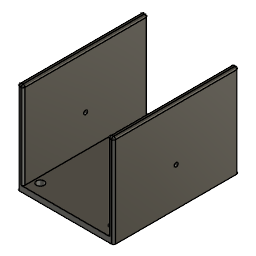
Servo Motor mount (Autodesk Fusion 360 design; units mm, degrees)
part number: 2026-06-29-17-08-25-141
Autodesk Fusion 360 part; units mm, degrees
sketch "Sketch1" plane through (0, 0, 0) normal (0, 0, 1) x (1, 0, 0)
  line L0 (0, 0) -> (50, 0)
  line L1 (50, 0) -> (50, 65)
  line L2 (50, 65) -> (0, 65)
  line L3 (0, 65) -> (0, 0)
  dimension "d1" = 50
  dimension "d2" = 65
  constraint horizontal L0
  constraint vertical L1
  constraint horizontal L2
  constraint vertical L3
  constraint coincident L0.start L3.end
  measures "d1" distance of L0.start L0.end
  measures "d2" distance of L0.start L2.end
extrude "Extrude1" add sketch "Sketch1" along normal blind 3
sketch "Sketch2" plane through (0, 0, 3) normal (0, 0, 1) x (-1, 0, 0)
  line L0 (0, -65) -> (0, 0)
  line L1 (0, 0) -> (-50, 0)
  line L2 (-50, 0) -> (-50, -65)
  line L3 (-50, -65) -> (0, -65)
  line L4 (0, -65) -> (-3, -65)
  line L5 (-3, -65) -> (-3, 0)
  line L6 (-3, 0) -> (0, 0)
  line L7 (0, 0) -> (0, -65)
  dimension "d5" = 65
  dimension "d6" = 50
  dimension "d7" = 3
  constraint horizontal L4
  constraint vertical L5
  constraint horizontal L6
  constraint vertical L7
  constraint coincident L1 L5.end
  constraint coincident L0.start L3.end
  measures "d5" distance of L0.start L0.end
  measures "d6" distance of L0.end L1.end
  measures "d7" distance of L0.start L4.end
extrude "Extrude2" add sketch "Sketch2" along normal blind 45 contours L0 L1 L3 L4 L5 L6 L7
sketch "Sketch3" plane through (0, 0, 3) normal (0, 0, 1) x (-1, 0, 0)
  line L0 (-3, -65) -> (-3, 0)
  line L1 (-3, 0) -> (-50, 0)
  line L2 (-50, 0) -> (-50, -65)
  line L3 (-50, -65) -> (-3, -65)
  line L4 (-50, -65) -> (-47, -65)
  line L5 (-47, -65) -> (-47, 0)
  line L6 (-47, 0) -> (-50, 0)
  line L7 (-50, 0) -> (-50, -65)
  dimension "d10" = 3
  constraint horizontal L4
  constraint vertical L5
  constraint horizontal L6
  constraint vertical L7
  constraint coincident L1 L5.end
  constraint coincident L2.end L3.start
  measures "d10" distance of L2.end L4.end
extrude "Extrude3" add sketch "Sketch3" along normal blind 45 contours L1 L2 L3 L4 L5 L6 L7
sketch "Sketch4" plane through (0, 0, 0) normal (-1, 0, 0) x (0, -1, 0)
  line L0 (-65, 0) -> (0, 0)
  line L1 (0, 0) -> (0, 48)
  line L2 (0, 48) -> (-65, 48)
  line L3 (-65, 48) -> (-65, 0)
  circle A0 centre (-32.5, 20) radius 1
  dimension "d14" = 2
  measures "d14" diameter of A0
extrude "Extrude4" cut sketch "Sketch4" against normal blind 51 contours A0
sketch "Sketch5" plane through (0, 0, 3) normal (0, 0, 1) x (-1, 0, 0)
  line L0 (-47, 0) -> (-47, -65)
  line L1 (-47, -65) -> (-3, -65)
  line L2 (-3, -65) -> (-3, 0)
  line L3 (-3, 0) -> (-47, 0)
  line L4 (0, 0) -> (-3, 0)
  circle A0 centre (-6, -59) radius 2
  circle A1 centre (-6, -6) radius 2
  circle A2 centre (-44, -6) radius 2
  circle A3 centre (-44, -59) radius 2
  dimension "d21" = 4
  dimension "d22" = 4
  dimension "d25" = 4
  dimension "d28" = 4
  constraint coincident L4.start origin
  constraint perpendicular L2 L4
  measures "d21" diameter of A0
  measures "d22" diameter of A1
  measures "d25" diameter of A2
  measures "d28" diameter of A3
extrude "Extrude5" cut sketch "Sketch5" against normal blind 5 contours A0 | A1 | A2 | A3
fillet "Fillet1" radius 1 4 edges at (50, 32.5, 48) (47, 32.5, 48) (3, 32.5, 48) (0, 32.5, 48)
fillet "Fillet2" radius 1 20 edges at (0, 65, 23.5) (0.2929, 65, 47.7071) (1.5, 65, 48) (2.7071, 65, 47.7071) (3, 65, 25) (47, 65, 25) (47.2929, 65, 47.7071) (48.5, 65, 48) (49.7071, 65, 47.7071) (50, 65, 23.5) (0, 0, 23.5) (0.2929, 0, 47.7071) (1.5, 0, 48) (2.7071, 0, 47.7071) (3, 0, 25) (47, 0, 25) (47.2929, 0, 47.7071) (48.5, 0, 48) (49.7071, 0, 47.7071) (50, 0, 23.5)
